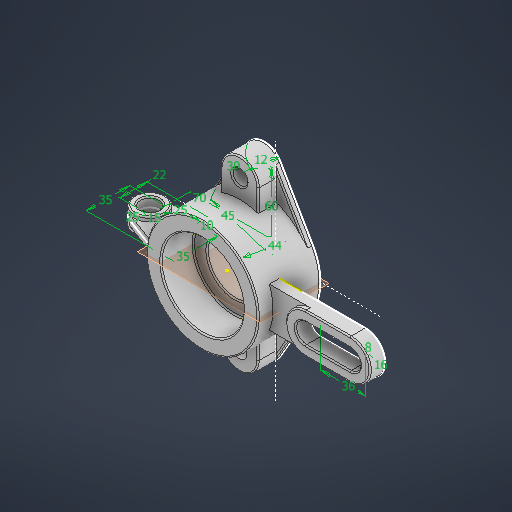
# Autodesk Inventor part: 부품1
Saved by Autodesk Inventor 2027.1 (Build 311270010, 270A)
## iProperties
Created: 2026-08-05
Part Number: 부품1
Material: 일반
Document SubType Name: Modeling
Designer: lkh06
Density: 1 g/cm^3
Appearance: 기본값
Author: lkh06
Autodesk Inventor part; units mm, degrees
ref_plane "YZ Plane" through (0, 0, 0) normal (1, 0, 0) x (0, 1, 0)
ref_plane "XZ Plane" through (0, 0, 0) normal (0, 1, 0) x (-1, 0, 0)
ref_plane "XY Plane" through (0, 0, 0) normal (0, 0, 1) x (1, 0, 0)
sketch "스케치1" plane through (0, 0, 0) normal (0, 0, 1) x (1, 0, 0)
  circle A0 centre (0, 0) radius 22
  line L0 (-87.457426, 0) -> (92.960648, 0) construction
  circle A1 centre (0, 60) radius 6
  circle A2 centre (0, -60) radius 6
  arc A3 (-45, 0) -> (-38.971143, -22.5) centre (0, 0) ccw
  arc A4 (12.990381, 67.5) -> (-12.990381, 67.5) centre (0, 60) ccw
  line L1 (-12.990381, 67.5) -> (-38.971143, 22.5)
  line L2 (12.990381, 67.5) -> (38.971143, 22.5)
  circle A5 centre (0, -60) radius 6
  arc A6 (-12.990381, -67.5) -> (12.990381, -67.5) centre (0, -60) ccw
  line L3 (-12.990381, -67.5) -> (-38.971143, -22.5)
  line L4 (12.990381, -67.5) -> (38.971143, -22.5)
  arc A7 (-38.971143, 22.5) -> (-45, 0) centre (0, 0) ccw
  arc A8 (-38.971143, -22.5) -> (38.971143, -22.5) centre (0, 0) ccw construction
  arc A9 (38.971143, 22.5) -> (-38.971143, 22.5) centre (0, 0) ccw construction
  arc A10 (38.971143, -22.5) -> (38.971143, 22.5) centre (0, 0) ccw
  line L5 (0, 75) -> (0, -75) construction
  dimension "d0" = 44
  dimension "d3" = 12
  dimension "d4" = 60
  dimension "d6" = 30
  dimension "d7" = 45
  constraints: 17 point on circle, 12 end point, 11 centre point, 7 symmetric about line, 4 coincident, 4 tangent, 2 point on line, 1 horizontal, 1 parallel, 1 vertical, 3 other
  measures "d0" diameter of A0
  measures "d3" diameter of A1
  measures "d4" distance of point (0, 0) A1.centre
  measures "d6" diameter of A4
  measures "d7" radius of A9
sketch "스케치2" plane through (0, 0, 0) normal (0, 0, 1) x (1, 0, 0)
  circle A0 centre (0, 0) radius 45
  circle A1 centre (0, 0) radius 33
  dimension "d10" = 90
  dimension "d11" = 66
  constraints: 2 centre point, 2 coincident
  measures "d10" diameter of A0
  measures "d11" diameter of A1
extrude "돌출1" add sketch "스케치1" along normal blind 5
extrude "돌출2" add sketch "스케치2" along normal blind 50
sketch "스케치3" plane through (0, 0, 5) normal (0, 0, 1) x (1, 0, 0)
  circle A0 centre (0, 0) radius 33
  circle A1 centre (0, 0) radius 22
  constraints: 2 centre point, 2 coincident
extrude "돌출3" add sketch "스케치3" along normal blind 19
sketch "스케치4" plane through (0, 0, 5) normal (0, 0, 1) x (1, 0, 0)
  circle A0 centre (0, -60) radius 6 construction
  arc A1 (-15, -60) -> (15, -60) centre (0, -60) ccw
  line L0 (15, -60) -> (15, -37.246804)
  line L1 (-15, -60) -> (-15, -37.246804)
  line L2 (-15, -37.246804) -> (15, -37.246804)
  arc A2 (15, -60) -> (-15, -60) centre (0, -60) ccw construction
  line L3 (125.953733, 0) -> (-121.771788, 0) construction
  circle A3 centre (0, 60) radius 6 construction
  arc A4 (15, 60) -> (-15, 60) centre (0, 60) ccw
  line L4 (15, 60) -> (15, 37.246804)
  line L5 (-15, 60) -> (-15, 37.246804)
  line L6 (-15, 37.246804) -> (15, 37.246804)
  arc A5 (-15, 60) -> (15, 60) centre (0, 60) ccw construction
  circle A6 centre (0, 60) radius 6
  circle A7 centre (0, -60) radius 6
  circle A8 centre (0, 60) radius 6 construction
  circle A9 centre (0, 60) radius 6
  point P0 (0, 0)
  point P1 (0, -75)
  dimension "d16" = 30
  dimension "d19" = 60
  constraints: 14 end point, 9 centre point, 9 point on circle, 9 symmetric about line, 6 coincident, 2 concentric, 2 tangent, 2 vertical, 1 horizontal, 1 perpendicular, 5 other
  measures "d16" distance of L1.end L0.end
  measures "d19" distance of A1.centre point (0, 0)
extrude "돌출4" add sketch "스케치4" along normal blind 15
sketch "스케치8" plane through (0, 0, 24) normal (0, 0, 1) x (1, 0, 0)
  circle A0 centre (0, 0) radius 33 construction
  line L0 (33, 0) -> (33, 103.401214) construction
  line L1 (33, 103.401214) -> (33, -77.851495) construction
  constraints: 4 end point, 2 vertical, 1 horizontal alignment, 1 point on line, 1 other
fillet "모깎기1" radius 1 1 edges at (-45, 0, 50)
fillet "모깎기2" radius 1 1 edges at (-33, 0, 50)
fillet "모깎기3" radius 1 1 edges at (-33, 0, 24)
fillet "모깎기4" radius 1 1 edges at (-22, 0, 24)
fillet "모깎기5" radius 1 1 edges at (-6, 60, 20)
fillet "모깎기6" radius 1 3 edges at (0, 75, 20) (-15, 51.2132, 20) (15, 51.2132, 20)
fillet "모깎기7" radius 1 3 edges at (0, -75, 20) (15, -51.2132, 20) (-15, -51.2132, 20)
fillet "모깎기8" radius 1 1 edges at (25.9808, -45, 5)
fillet "모깎기9" radius 1 1 edges at (25.9808, 45, 5)
fillet "모깎기10" radius 1 1 edges at (-25.9808, 45, 5)
fillet "모깎기11" radius 1 1 edges at (-25.9808, -45, 5)
fillet "모깎기12" radius 1 8 edges at (-45, 0, 0) (-25.9808, -45, 0) (0, -75, 0) (25.9808, -45, 0) (45, 0, 0) (25.9808, 45, 0) (0, 75, 0) (-25.9808, 45, 0)
fillet "모깎기13" radius 1 1 edges at (-6, 60, 0)
fillet "모깎기14" radius 1 1 edges at (-6, -60, 0)
ref_plane "작업 평면3" through (-87.457426, 0, 0) normal (0, 1, 0) x (1, 0, 0)
sketch "스케치11" plane through (-87.457426, 0, 0) normal (0, 1, 0) x (1, 0, 0)
  point P0 (87.457426, 0)
sketch "스케치12" plane through (-87.457426, 0, 0) normal (0, 1, 0) x (1, 0, 0)
  circle A0 centre (17.457426, -22) radius 7.5
  line L0 (75.333071, 0) -> (99.581782, 0)
  line L1 (43.457426, 0) -> (49.352309, 0)
  circle A1 centre (17.457426, -22) radius 12.5
  line L2 (17.457426, -9.5) -> (42.457426, -9.5)
  line L3 (42.457426, -1) -> (42.457426, -49)
  line L4 (13.147346, -33.733423) -> (42.457426, -44.5)
  line L5 (42.457426, -44.5) -> (52.457426, -44.5)
  line L6 (52.457426, -44.5) -> (52.457426, -9.5)
  line L7 (52.457426, -9.5) -> (42.457426, -9.5)
  point P0 (87.457426, 0)
  point P1 (87.457426, 0)
  dimension "d57" = 15
  dimension "d58" = 70
  dimension "d59" = 22
  dimension "d60" = 25
  dimension "d62" = 25
  dimension "d64" = 35
  dimension "d67" = 10
  dimension "d68" = 35
  constraints: 10 end point, 2 centre point, 2 horizontal, 2 point on circle, 2 point on line, 1 coincident, 1 midpoint, 1 parallel, 1 perpendicular, 1 tangent
  measures "d57" diameter of A0
  measures "d58" horizontal distance of A0.centre point (87.457, 0)
  measures "d59" distance from line of L1 A0.centre
  measures "d60" diameter of A1
  measures "d62" distance of L2.start L2.end
  measures "d64" vertical distance of L2.start L4.end
  measures "d67" distance of L7.end L6.end
  measures "d68" distance of L5.end L6.end
extrude "돌출7" add sketch "스케치12" along normal mid plane 8 contours A1 L2 L3 L4 | L7 L6 L5 L3
extrude "돌출8" add sketch "스케치12" along normal mid plane 15 contours A1
fillet "모깎기15" radius 1 1 edges at (-82.5, 7.5, 22)
fillet "모깎기16" radius 1 1 edges at (-77.5, 7.5, 22)
fillet "모깎기17" radius 1 1 edges at (-82.5, -7.5, 22)
fillet "모깎기18" radius 1 1 edges at (-77.5, -7.5, 22)
sketch "스케치13" plane through (-87.457426, 0, 0) normal (0, 1, 0) x (1, 0, 0)
  line L0 (120.457426, -49) -> (120.457426, -25)
  line L1 (120.457426, -38) -> (154.457426, -38)
  line L2 (154.457426, -38) -> (154.457426, -30)
  line L3 (154.457426, -30) -> (120.457426, -30)
  line L4 (120.457426, -30) -> (120.457426, -38)
  line L5 (100.447807, -1) -> (74.467045, -1)
  line L6 (125.562544, 0) -> (131.457426, 0)
  point P0 (87.457426, 0)
  point P1 (87.457426, -1)
  dimension "d75" = 8
  dimension "d76" = 67
  dimension "d77" = 30
  constraints: 8 end point, 2 parallel, 1 horizontal, 1 midpoint, 1 perpendicular, 1 point on line
  measures "d75" distance of L2.end L1.end
  measures "d76" distance from line of point (87.457, -1) L2
  measures "d77" distance between parallel lines of L6 L3
extrude "돌출9" add sketch "스케치13" along normal mid plane 32
sketch "스케치14" plane through (67, 16, 30) normal (0, 0, -1) x (-1, 0, 0)
  line L0 (0, -32) -> (24.940518, -32)
  line L1 (5.086706, -32) -> (-8, -32)
  arc A0 (-8, -32) -> (-8, 0) centre (-8, -16) ccw
  line L2 (0, 0) -> (0, -32)
  line L3 (-8, 0) -> (6.248366, 0)
  line L4 (24.940518, 0) -> (0, 0)
  line L5 (0, 0) -> (24.940518, 0)
  arc A1 (-8, -24) -> (-8, -8) centre (-8, -16) ccw
  arc A2 (-44, -8) -> (-44, -24) centre (-44, -16) ccw
  arc A3 (-44, 0) -> (-44, -32) centre (-44, -16) ccw
  line L6 (-44, -32) -> (-8, -32)
  line L7 (-44, 0) -> (-8, 0)
  line L8 (-44, -24) -> (-8, -24)
  line L9 (-44, -8) -> (-8, -8)
  point P0 (67, -16)
  point P1 (0, -16)
  point P2 (0, -2.143594)
  point P3 (0, -29.856406)
  dimension "d89" = 8
  dimension "d90" = 36
  dimension "d91" = 16
  constraints: 12 end point, 9 point on circle, 8 tangent, 4 centre point, 2 coincident, 2 collinear, 2 equal radius, 2 parallel, 2 point on line, 1 midpoint
  measures "d89" radius of A2
  measures "d90" distance of A2.centre A0.centre
  measures "d91" radius of A3
extrude "돌출10" add sketch "스케치14" against normal blind 12 contours L6 A3 L7 A0 L2 | L2 A0
extrude "돌출11" add sketch "스케치14" against normal blind 8 contours A0 L3 L2
extrude "돌출12" add sketch "스케치14" against normal blind 8 contours L1 A0 L2
fillet "모깎기19" radius 1 4 edges at (119, 0, 42) (93, -8, 42) (67, 0, 42) (93, 8, 42)
fillet "모깎기20" radius 1 4 edges at (59, 0, 42) (93, -16, 42) (127, 0, 42) (93, 16, 42)
